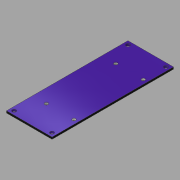
# Autodesk Inventor part: STARduino layout
Saved by Autodesk Inventor 2017 (Build 210142000, 142)
## iProperties
Created: 2017-01-15
Part Number: STARduino layout
Material: Generic
Document SubType Name: Modeling
Designer: qupec
Density: 1 g/cm^3
Appearance: Default
Author: qupec
Autodesk Inventor part; units mm, degrees
ref_plane "YZ Plane" through (0, 0, 0) normal (1, 0, 0) x (0, 1, 0)
ref_plane "XZ Plane" through (0, 0, 0) normal (0, 1, 0) x (-1, 0, 0)
ref_plane "XY Plane" through (0, 0, 0) normal (0, 0, 1) x (1, 0, 0)
sketch "Sketch1" plane through (0, 0, 0) normal (0, 1, 0) x (-1, 0, 0)
  line L0 (19.05, 50.8) -> (6.35, 50.8)
  line L1 (6.35, -50.8) -> (19.05, -50.8)
  line L2 (19.05, -50.8) -> (19.05, 50.8)
  line L3 (6.35, 50.8) -> (-19.05, 50.8)
  line L4 (-19.05, 50.8) -> (-19.05, -50.8)
  line L5 (-19.05, -50.8) -> (6.35, -50.8)
  line L6 (6.35, -50.8) -> (6.35, -50.8)
  line L7 (6.35, 50.8) -> (6.35, 50.8)
  point P0 (0, 0)
  dimension "d0" = 101.6
  dimension "d2" = 101.6
  dimension "d3" = 0
  dimension "d4" = 12.7
  dimension "d5" = 25.4
  dimension "d6" = 0
  dimension "d7" = 50.8
  dimension "d8" = 38.1
  dimension "d9" = 19.05
  dimension "d10" = 12.7
  constraints: 16 end point, 4 parallel, 2 horizontal, 1 perpendicular
  measures "d0" distance of L1.end L0.start
  measures "d2" distance of L3.end L4.end
  measures "d3" distance between parallel lines of L0 L3
  measures "d4" distance of L0.start L0.end
  measures "d5" distance of L3.start L3.end
  measures "d6" distance of L5.end L1.start
  measures "d7" distance from line of point (0, 0) L3
  measures "d8" distance of L4.end L1.end
  measures "d9" distance from line of point (0, 0) L2
  measures "d10" distance of L1.start L1.end
extrude "Extrusion1" add sketch "Sketch1" along normal blind 1.651
sketch "Sketch2" plane through (0, 1.651, 0) normal (0, 1, 0) x (1, 0, 0)
  circle A0 centre (-15.875, -47.625) radius 1.5875
  circle A1 centre (15.875, -47.625) radius 1.5875
  circle A2 centre (-15.875, 47.625) radius 1.5875
  circle A3 centre (15.875, 47.625) radius 1.5875
  line L0 (19.05, 50.8) -> (-19.05, 50.8) projected
  line L1 (-19.05, 50.8) -> (-19.05, -50.8) projected
  line L2 (19.05, -50.8) -> (19.05, 50.8) projected
  line L3 (-19.05, -50.8) -> (19.05, -50.8) projected
  point P0 (0, 0)
  point P1 (-6.35, 38.1)
  dimension "d13" = 3.175
  dimension "d14" = 3.175
  dimension "d15" = 3.175
  dimension "d16" = 3.175
  dimension "d17" = 3.175
  dimension "d18" = 3.175
  dimension "d19" = 3.175
  dimension "d20" = 3.175
  dimension "d21" = 3.175
  dimension "d22" = 3.175
  dimension "d23" = 3.175
  dimension "d27" = 3.175
  constraints: 4 centre point, 1 other
  measures "d13" diameter of A2
  measures "d14" diameter of A3
  measures "d15" diameter of A0
  measures "d16" diameter of A1
  measures "d18" distance from line of L1 A2.centre
  measures "d19" distance from line of L2 A3.centre
  measures "d21" distance from line of L2 A1.centre
  measures "d22" distance from line of L3 A1.centre
  measures "d23" distance from line of L3 A0.centre
  measures "d27" distance from line of L1 A0.centre
extrude "Extrusion2" cut sketch "Sketch2" against normal through all contours A0 | A1 | A2 | A3
sketch "Sketch3" plane through (0, 1.651, 0) normal (0, 1, 0) x (1, 0, 0)
  circle A0 centre (-7.45, 29) radius 1.375
  circle A1 centre (15.55, 29) radius 1.375
  circle A2 centre (-7.45, -29) radius 1.375
  circle A3 centre (15.55, -29) radius 1.375
  line L0 (-19.05, -50.8) -> (19.05, -50.8) projected
  line L1 (19.05, 50.8) -> (-19.05, 50.8) projected
  line L2 (-19.05, 50.8) -> (-19.05, -50.8) projected
  line L3 (19.05, -50.8) -> (19.05, 50.8) projected
  point P0 (0, 0)
  dimension "d28" = 2.75
  dimension "d29" = 2.75
  dimension "d30" = 2.75
  dimension "d31" = 2.75
  dimension "d32" = 23
  dimension "d33" = 23
  dimension "d34" = 58
  dimension "d35" = 101.6
  dimension "d36" = 29
  dimension "d39" = 0
  dimension "d40" = 0
  dimension "d41" = 58
  dimension "d44" = 3.5
  constraints: 4 centre point
  measures "d28" diameter of A0
  measures "d29" diameter of A1
  measures "d30" diameter of A2
  measures "d31" diameter of A3
  measures "d32" distance of A1.centre A0.centre
  measures "d33" distance of A3.centre A2.centre
  measures "d34" distance of A2.centre A0.centre
  measures "d35" distance between parallel lines of L0 L1
  measures "d36" vertical distance of point (0, 0) A2.centre
  measures "d39" horizontal distance of A3.centre A1.centre
  measures "d40" horizontal distance of A2.centre A0.centre
  measures "d41" distance of A3.centre A1.centre
  measures "d44" distance from line of L3 A1.centre
extrude "Extrusion3" cut sketch "Sketch3" against normal through all contours A0 | A1 | A2 | A3
equation "\"d0\" = d2"
equation "\"d6\" = d3"
equation "\"d7\" = 0.5 * d2"
equation "\"d9\" = 0.5 * d8"
equation "\"d10\" = d4"
equation "\"d14\" = d13"
equation "\"d15\" = d13"
equation "\"d16\" = d13"
equation "\"d19\" = d18"
equation "\"d20\" = d17"
equation "\"d21\" = d19"
equation "\"d22\" = d17"
equation "\"d23\" = d17"
equation "\"d27\" = d21"
equation "\"d29\" = d28"
equation "\"d30\" = d28"
equation "\"d31\" = d28"
equation "\"d32\" = d33"
equation "\"d36\" = 0.5 * d34"
equation "\"d41\" = d34"
body "Solid1"
